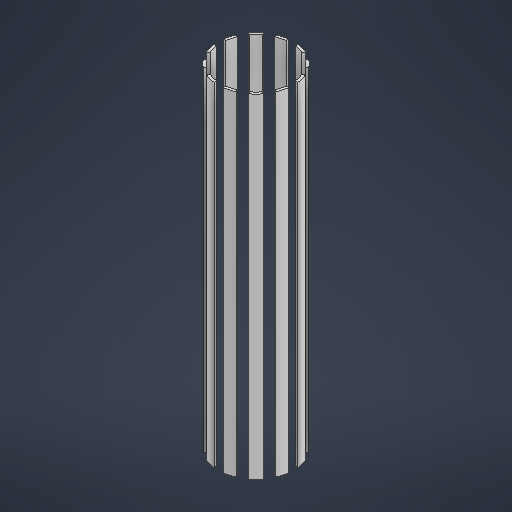
# Autodesk Inventor part: bandstoproller
Saved by Autodesk Inventor 2026.1 (Build 301233000, 233)
## iProperties
Created: 2025-08-08
Part Number: bandstoproller
Material: Generic
Document SubType Name: Modeling
Designer: roejo
Density: 1 g/cm^3
Appearance: Default
Author: roejo
Autodesk Inventor part; units mm, degrees
ref_plane "YZ Plane" through (0, 0, 0) normal (1, 0, 0) x (0, 1, 0)
ref_plane "XZ Plane" through (0, 0, 0) normal (0, 1, 0) x (-1, 0, 0)
ref_plane "XY Plane" through (0, 0, 0) normal (0, 0, 1) x (1, 0, 0)
sketch "Sketch1" plane through (0, 0, 0) normal (0, 1, 0) x (-1, 0, 0)
  circle A0 centre (0, 0) radius 23.8125
  dimension "d0" = 47.625
  constraints: 1 centre point, 1 coincident
  measures "d0" diameter of A0
extrude "Extrusion1" add sketch "Sketch1" along normal blind 211.0232
sketch "Sketch2" plane through (0, 211.0232, 0) normal (0, 1, 0) x (1, 0, 0)
  circle A0 centre (0, 0) radius 22.225
  dimension "d3" = 44.45
  constraints: 1 centre point, 1 coincident
  measures "d3" diameter of A0
extrude "Extrusion2" cut sketch "Sketch2" against normal through all
sketch "Sketch3" plane through (0, 211.0232, 0) normal (0, 1, 0) x (1, 0, 0)
  line L0 (-25.4, -2.8575) -> (-20.32, -2.8575)
  line L1 (-20.32, -2.8575) -> (-20.32, 2.8575)
  line L2 (-20.32, 2.8575) -> (-25.4, 2.8575)
  line L3 (-25.4, 2.8575) -> (-25.4, -2.8575)
  line L4 (-20.5683, -15.1747) -> (-16.1689, -12.6347)
  line L5 (-16.1689, -12.6347) -> (-19.0264, -7.6853)
  line L6 (-19.0264, -7.6853) -> (-23.4258, -10.2253)
  line L7 (-23.4258, -10.2253) -> (-20.5683, -15.1747)
  line L8 (-10.2253, -23.4258) -> (-7.6853, -19.0264)
  line L9 (-7.6853, -19.0264) -> (-12.6347, -16.1689)
  line L10 (-12.6347, -16.1689) -> (-15.1747, -20.5683)
  line L11 (-15.1747, -20.5683) -> (-10.2253, -23.4258)
  line L12 (2.8575, -25.4) -> (2.8575, -20.32)
  line L13 (2.8575, -20.32) -> (-2.8575, -20.32)
  line L14 (-2.8575, -20.32) -> (-2.8575, -25.4)
  line L15 (-2.8575, -25.4) -> (2.8575, -25.4)
  line L16 (15.1747, -20.5683) -> (12.6347, -16.1689)
  line L17 (12.6347, -16.1689) -> (7.6853, -19.0264)
  line L18 (7.6853, -19.0264) -> (10.2253, -23.4258)
  line L19 (10.2253, -23.4258) -> (15.1747, -20.5683)
  line L20 (23.4258, -10.2253) -> (19.0264, -7.6853)
  line L21 (19.0264, -7.6853) -> (16.1689, -12.6347)
  line L22 (16.1689, -12.6347) -> (20.5683, -15.1747)
  line L23 (20.5683, -15.1747) -> (23.4258, -10.2253)
  line L24 (25.4, 2.8575) -> (20.32, 2.8575)
  line L25 (20.32, 2.8575) -> (20.32, -2.8575)
  line L26 (20.32, -2.8575) -> (25.4, -2.8575)
  line L27 (25.4, -2.8575) -> (25.4, 2.8575)
  line L28 (20.5683, 15.1747) -> (16.1689, 12.6347)
  line L29 (16.1689, 12.6347) -> (19.0264, 7.6853)
  line L30 (19.0264, 7.6853) -> (23.4258, 10.2253)
  line L31 (23.4258, 10.2253) -> (20.5683, 15.1747)
  line L32 (10.2253, 23.4258) -> (7.6853, 19.0264)
  line L33 (7.6853, 19.0264) -> (12.6347, 16.1689)
  line L34 (12.6347, 16.1689) -> (15.1747, 20.5683)
  line L35 (15.1747, 20.5683) -> (10.2253, 23.4258)
  line L36 (-2.8575, 25.4) -> (-2.8575, 20.32)
  line L37 (-2.8575, 20.32) -> (2.8575, 20.32)
  line L38 (2.8575, 20.32) -> (2.8575, 25.4)
  line L39 (2.8575, 25.4) -> (-2.8575, 25.4)
  line L40 (-15.1747, 20.5683) -> (-12.6347, 16.1689)
  line L41 (-12.6347, 16.1689) -> (-7.6853, 19.0264)
  line L42 (-7.6853, 19.0264) -> (-10.2253, 23.4258)
  line L43 (-10.2253, 23.4258) -> (-15.1747, 20.5683)
  line L44 (-23.4258, 10.2253) -> (-19.0264, 7.6853)
  line L45 (-19.0264, 7.6853) -> (-16.1689, 12.6347)
  line L46 (-16.1689, 12.6347) -> (-20.5683, 15.1747)
  line L47 (-20.5683, 15.1747) -> (-23.4258, 10.2253)
  circle A0 centre (0, 0) radius 23.8125 projected
  point P0 (-30.1625, 0)
  point P1 (-26.1215, -15.0812)
  point P2 (-15.0813, -26.1215)
  point P3 (0, -30.1625)
  point P4 (15.0812, -26.1215)
  point P5 (26.1215, -15.0813)
  point P6 (30.1625, 0)
  point P7 (26.1215, 15.0812)
  point P8 (15.0813, 26.1215)
  point P9 (0, 30.1625)
  point P10 (-15.0812, 26.1215)
  point P11 (-26.1215, 15.0813)
  dimension "d13" = 360
  dimension "d16" = 20.32
  constraints: 96 end point, 2 parallel, 1 horizontal, 1 perpendicular, 109 other
  measures "d16" distance from line of A0.centre L1
extrude "Extrusion3" cut sketch "Sketch3" against normal through all contours L3 L2 A0 L0 | A0 L2 L1 L0 | A0 L4 L7 L6 | L6 L5 L4 A0 | A0 L46 L45 L44 | L44 L47 L46 A0 | A0 L8 L11 L10 | L10 L9 L8 A0 | A0 L42 L41 L40 | L40 L43 L42 A0 | A0 L12 L15 L14 | L14 L13 L12 A0 | A0 L38 L37 L36 | L36 L39 L38 A0 | A0 L16 L19 L18 | L18 L17 L16 A0 | A0 L34 L33 L32 | L32 L35 L34 A0 | A0 L20 L23 L22 | L22 L21 L20 A0 | A0 L30 L29 L28 | L28 L31 L30 A0 | A0 L24 L27 L26 | L26 L25 L24 A0
body "Solid1"
